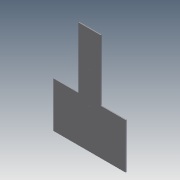
# Autodesk Inventor part: front
Saved by Autodesk Inventor 2011 (Build 150239000, 239)
## iProperties
Created: 2011-10-30
Part Number: front
Document SubType Name: Modeling
Designer: Matthew
Density: 1 g/cm^3
Author: Matthew
Autodesk Inventor part; units mm, degrees
ref_plane "YZ Plane" through (0, 0, 0) normal (1, 0, 0) x (0, 1, 0)
ref_plane "XZ Plane" through (0, 0, 0) normal (0, 1, 0) x (-1, 0, 0)
ref_plane "XY Plane" through (0, 0, 0) normal (0, 0, 1) x (1, 0, 0)
sketch "Sketch1" plane through (0, 0, 0) normal (0, 0, 1) x (1, 0, 0)
  line L0 (-73.5219, 27.2789) -> (440.7773, 27.2789)
  line L1 (440.7773, 27.2789) -> (440.7773, -861.7211)
  line L2 (440.7773, -861.7211) -> (-73.5219, -861.7211)
  line L3 (-73.5219, -861.7211) -> (-73.5219, 27.2789)
  point P0 (0, 0)
  dimension "d0" = 514.2992
  dimension "d1" = 889
  constraints: 8 end point, 2 parallel, 1 horizontal, 1 perpendicular
  measures "d0" distance of L1.end L2.end
  measures "d1" distance of L0.end L1.end
extrude "Extrusion1" add sketch "Sketch1" along normal blind 6.35
sketch "Sketch3" plane through (0, 0, 6.35) normal (0, 0, 1) x (1, 0, 0)
  line L0 (-73.5219, 27.2789) -> (104.2781, 27.2789)
  line L1 (104.2781, 27.2789) -> (104.2781, -433.4771)
  line L2 (104.2781, -433.4771) -> (-73.5219, -433.4771)
  line L3 (-73.5219, -433.4771) -> (-73.5219, 27.2789)
  line L4 (440.7773, 27.2789) -> (262.9773, 27.2789)
  line L5 (262.9773, 27.2789) -> (262.9773, -433.4771)
  line L6 (262.9773, -433.4771) -> (440.7773, -433.4771)
  line L7 (440.7773, -433.4771) -> (440.7773, 27.2789)
  point P0 (0, 0)
  dimension "d4" = 177.8
  dimension "d5" = 460.756
  dimension "d6" = 177.8
  dimension "d7" = 460.756
  constraints: 16 end point, 4 parallel, 2 horizontal, 2 perpendicular
  measures "d4" distance of L1.end L2.end
  measures "d5" distance of L0.end L1.end
  measures "d6" distance of L6.end L5.end
  measures "d7" distance of L5.end L4.end
extrude "Extrusion2" cut sketch "Sketch3" against normal blind 25.4
sketch "Sketch4" plane through (104.2781, 27.2789, 0) normal (0, 1, 0) x (1, 0, 0)
  line L0 (0, 0) -> (0, -6.35) projected
  line L1 (0, -6.35) -> (158.6992, -6.35) projected
  line L2 (158.6992, -6.35) -> (158.6992, 0) projected
  line L3 (0, 0) -> (158.6992, 0) projected
  point P0 (-104.2781, 0)
extrude "Extrusion3" add sketch "Sketch4" along normal blind 6.35
sketch "Sketch5" plane through (104.2781, 33.6289, 0) normal (0, 1, 0) x (1, 0, 0)
  line L0 (0, 0) -> (158.6992, 0) projected
  line L1 (0, -6.35) -> (0, 0) projected
  line L2 (158.6992, -6.35) -> (0, -6.35) projected
  line L3 (158.6992, 0) -> (158.6992, -6.35) projected
  point P0 (-104.2781, 0)
extrude "Extrusion4" cut sketch "Sketch5" against normal blind 6.35
sketch "Sketch6" plane through (104.2781, 27.2789, 0) normal (0, 1, 0) x (1, 0, 0)
  line L0 (0, -6.35) -> (0, 0) projected
  line L1 (158.6992, -6.35) -> (0, -6.35) projected
  line L2 (158.6992, 0) -> (158.6992, -6.35) projected
  line L3 (0, 0) -> (158.6992, 0) projected
  point P0 (-104.2781, 0)
extrude "Extrusion5" add sketch "Sketch6" along normal blind 6.35
sketch "Sketch7" plane through (0, 0, 0) normal (0, 0, -1) x (-1, 0, 0)
  line L0 (-440.7773, -861.7211) -> (73.5219, -861.7211) projected
  line L1 (-104.2781, 33.6289) -> (-262.9773, 33.6289) projected
  line L2 (-183.6277, -861.7211) -> (-183.6277, -362.9159)
  circle A0 centre (-183.6277, -362.9159) radius 2.3495
  point P0 (0, 0)
  dimension "d16" = 498.8052
  dimension "d17" = 4.699
  constraints: 2 end point, 1 centre point, 1 coincident, 1 midpoint, 1 perpendicular
  measures "d16" distance of L2.start L2.end
  measures "d17" diameter of A0
extrude "Extrusion6" cut sketch "Sketch7" against normal blind 25.4
sketch "Sketch8" plane through (0, 0, 0) normal (0, 0, -1) x (-1, 0, 0)
  circle A0 centre (-183.6277, -362.9159) radius 2.3495 projected
  line L0 (-104.2781, 33.6289) -> (-262.9773, 33.6289) projected
  line L1 (-183.6277, -362.9159) -> (-183.6277, -593.4209)
  circle A1 centre (-183.6277, -593.4209) radius 2.3495
  point P0 (0, 0)
  dimension "d20" = 230.505
  dimension "d21" = 4.699
  constraints: 2 end point, 1 centre point, 1 coincident, 1 perpendicular
  measures "d20" distance of L1.start L1.end
  measures "d21" diameter of A1
extrude "Extrusion7" cut sketch "Sketch8" against normal blind 25.4 contours A1
sketch "Sketch9" plane through (0, 0, 0) normal (0, 0, -1) x (-1, 0, 0)
  circle A0 centre (-183.6277, -593.4209) radius 2.3495 projected
  circle A1 centre (-183.6277, -362.9159) radius 2.3495 projected
  line L0 (-104.2781, 33.6289) -> (-262.9773, 33.6289) projected
  line L1 (-183.6277, 33.6289) -> (-183.6277, -347.3711)
  circle A2 centre (-183.6277, -347.3711) radius 2.3495
  line L2 (-183.6277, -347.3711) -> (-183.6277, -362.9159)
  line L3 (-183.6277, -593.4209) -> (-183.6277, -577.8761)
  circle A3 centre (-183.6277, -577.8761) radius 2.3495
  point P0 (0, 0)
  dimension "d24" = 381
  dimension "d25" = 15.5448
  constraints: 6 end point, 2 centre point, 2 coincident, 2 collinear, 1 midpoint, 1 perpendicular
  measures "d24" distance of L1.start L1.end
  measures "d25" distance of L3.start L3.end
extrude "Extrusion8" cut sketch "Sketch9" against normal blind 25.4 contours A2 L2 L1 | L1 L2 A2 | A3
sketch "Sketch10" plane through (0, 0, 0) normal (0, 0, -1) x (-1, 0, 0)
  circle A0 centre (-183.6277, -593.4209) radius 2.3495 projected
  circle A1 centre (-183.6277, -362.9159) radius 2.3495 projected
  point P0 (0, 0)
extrude "Extrusion9" add sketch "Sketch10" against normal blind 6.35
sketch "Sketch11" plane through (0, 0, 6.35) normal (0, 0, 1) x (1, 0, 0)
  line L0 (104.2781, -433.4771) -> (-73.5219, -433.4771) projected
  line L1 (-73.5219, -861.7211) -> (-73.5219, -433.4771) projected
  line L2 (440.7773, -861.7211) -> (-73.5219, -861.7211) projected
  line L3 (440.7773, -433.4771) -> (440.7773, -861.7211) projected
  line L4 (262.9773, 33.6289) -> (104.2781, 33.6289) projected
  line L5 (49.7648, -433.4771) -> (49.7648, -750.9771)
  line L6 (49.7648, -750.9771) -> (49.7648, -757.3271)
  line L7 (49.7648, -757.3271) -> (-73.5219, -757.3271)
  line L8 (49.7648, -757.3271) -> (440.7773, -757.3271)
  point P0 (0, 0)
  dimension "d30" = 317.5
  dimension "d31" = 6.35
  constraints: 8 end point, 3 perpendicular, 3 point on line, 1 collinear
  measures "d30" distance of L5.start L5.end
  measures "d31" distance of L5.end L6.end
extrude "Extrusion10" cut sketch "Sketch11" against normal blind 6.35 contours L7 L8 L3 L2 L1
sketch "Sketch12" plane through (0, 0, 0) normal (0, 0, -1) x (-1, 0, 0)
  line L0 (-440.7773, -433.4771) -> (-440.7773, -757.3271) projected
  circle A0 centre (-183.6277, -577.8761) radius 2.3495 projected
  circle A1 centre (-183.6277, -347.3711) radius 2.3495 projected
  line L1 (-183.6277, -347.3711) -> (-183.6277, -249.3271)
  line L2 (-183.6277, -577.8761) -> (-183.6277, -479.8321)
  circle A2 centre (-183.6277, -479.8321) radius 2.3495
  circle A3 centre (-183.6277, -249.3271) radius 2.3495
  point P0 (0, 0)
  dimension "d34" = 98.044
  dimension "d35" = 98.044
  constraints: 4 end point, 2 centre point, 2 coincident, 1 collinear, 1 parallel
  measures "d34" distance of L1.start L1.end
  measures "d35" distance of L2.start L2.end
extrude "Extrusion11" cut sketch "Sketch12" against normal blind 6.35 contours A2 | A3
sketch "Sketch13" plane through (0, 0, 0) normal (0, 0, -1) x (-1, 0, 0)
  circle A0 centre (-183.6277, -577.8761) radius 2.3495 projected
  circle A1 centre (-183.6277, -347.3711) radius 2.3495 projected
  point P0 (0, 0)
extrude "Extrusion12" add sketch "Sketch13" against normal blind 6.35
sketch "Sketch14" plane through (0, 0, 6.35) normal (0, 0, 1) x (1, 0, 0)
  line L0 (262.9773, -433.4771) -> (262.9773, 33.6289) projected
  line L1 (104.2781, 33.6289) -> (262.9773, 33.6289)
  line L2 (262.9773, 33.6289) -> (262.9773, 14.5789)
  line L3 (262.9773, 14.5789) -> (104.2781, 14.5789)
  line L4 (104.2781, 14.5789) -> (104.2781, 33.6289)
  point P0 (0, 0)
  dimension "d40" = 19.05
  constraints: 8 end point, 2 parallel, 1 horizontal, 1 perpendicular, 1 point on line
  measures "d40" distance of L1.end L2.end
extrude "Extrusion13" cut sketch "Sketch14" against normal blind 25.4
sketch "Sketch15" plane through (0, 0, 6.35) normal (0, 0, 1) x (1, 0, 0)
  line L0 (262.9773, -433.4771) -> (262.9773, 14.5789) projected
  line L1 (104.2781, 14.5789) -> (262.9773, 14.5789)
  line L2 (262.9773, 14.5789) -> (262.9773, 1.8789)
  line L3 (262.9773, 1.8789) -> (104.2781, 1.8789)
  line L4 (104.2781, 1.8789) -> (104.2781, 14.5789)
  point P0 (0, 0)
  dimension "d43" = 12.7
  constraints: 8 end point, 2 parallel, 1 horizontal, 1 perpendicular, 1 point on line
  measures "d43" distance of L1.end L2.end
extrude "Extrusion14" cut sketch "Sketch15" against normal blind 25.4
body "Solid1"
